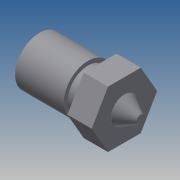
# Autodesk Inventor part: nozzle
Saved by Autodesk Inventor 2013 (Build 170138000, 138)
## iProperties
Created: 2017-04-01
Part Number: nozzle
Material: Generic
Document SubType Name: Modeling
Designer: employee
Density: 1 g/cm^3
Author: employee
Autodesk Inventor part; units mm, degrees
ref_plane "YZ Plane" through (0, 0, 0) normal (1, 0, 0) x (0, 1, 0)
ref_plane "XZ Plane" through (0, 0, 0) normal (0, 1, 0) x (-1, 0, 0)
ref_plane "XY Plane" through (0, 0, 0) normal (0, 0, 1) x (1, 0, 0)
sketch "Sketch1" plane through (0, 0, 0) normal (0, 0, 1) x (1, 0, 0)
  line L0 (0, 0) -> (-10.5, 0)
  line L1 (-10.5, 0) -> (-10.5, -3)
  line L2 (-10.5, -3) -> (-4.5, -3)
  line L3 (-4.5, -3) -> (-4.5, -2.5)
  line L4 (-4.5, -2.5) -> (-3, -2.5)
  line L5 (-3, -2.5) -> (-3, -10)
  line L6 (-3, -10) -> (0, -10)
  line L7 (0, -10) -> (0, -1.6547)
  line L8 (0, -1.6547) -> (2, -0.5)
  line L9 (2, -0.5) -> (2, 0)
  line L10 (2, 0) -> (0, 0)
  dimension "d0" = 0.5
  dimension "d3" = 3
  dimension "d5" = 2.5
  dimension "d6" = 10
  dimension "d7" = 10.5
  dimension "d8" = 2
  dimension "d9" = 30
  dimension "d10" = 7.5
  dimension "d11" = 6
  constraints: 22 end point, 7 parallel, 1 collinear, 1 horizontal, 1 perpendicular, 1 vertical alignment
  measures "d0" distance of L8.end L9.end
  measures "d3" distance of L0.end L1.end
  measures "d5" distance between parallel lines of L0 L4
  measures "d6" distance between parallel lines of L6 L10
  measures "d7" distance between parallel lines of L7 L1
  measures "d8" distance from line of L9.end L7
  measures "d9" angle of L8 L10
  measures "d10" distance between parallel lines of L5 L1
  measures "d11" distance of L1.end L2.end
revolve "Revolution1" add sketch "Sketch1" angle 360 about axis through (0, 0, 0) along (-1, 0, 0)
sketch "Sketch2" plane through (0, 0, 0) normal (1, 0, 0) x (0, 0, -1)
  circle A0 centre (0, 0) radius 10 projected
  circle A1 centre (0, 0) radius 1.6547 projected
  line L0 (0, 4.0415) -> (3.5, 2.0207)
  line L1 (3.5, 2.0207) -> (3.5, -2.0207)
  line L2 (3.5, -2.0207) -> (0, -4.0415)
  line L3 (0, -4.0415) -> (-3.5, -2.0207)
  line L4 (-3.5, -2.0207) -> (-3.5, 2.0207)
  line L5 (-3.5, 2.0207) -> (0, 4.0415)
  dimension "d13" = 7
  constraints: 12 end point, 1 coincident, 1 vertical, 13 other
  measures "d13" distance between parallel lines of L1 L4
extrude "Extrusion1" cut sketch "Sketch2" against normal up to surface (3 mm away) contours A0
body "Solid1"
